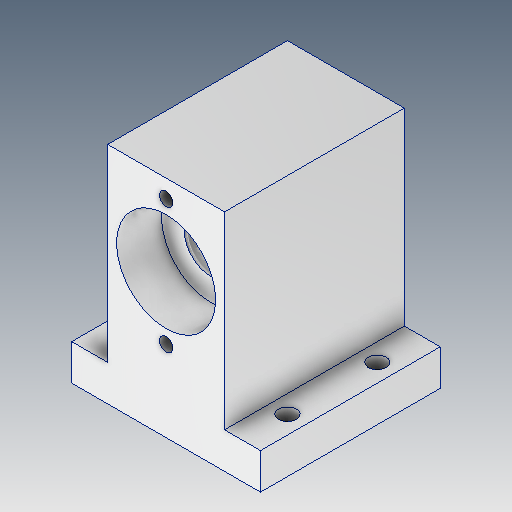
# Autodesk Inventor part: Soporte de tuerca de mesa
Saved by Autodesk Inventor 2020.3 (Build 243373000, 373)
## iProperties
Created: 2020-05-16
Part Number: Soporte de tuerca de mesa
Material: Aluminum 6061
Document SubType Name: Modeling
Designer: Pipi
Density: 2.7 g/cm^3
Appearance: Aluminum - Flat
Mass: 118.391 g
Surface Area: 121.696 cm^2
Volume: 43.8487 cm^3
Author: Pipi
Autodesk Inventor part; units mm, degrees
ref_plane "YZ Plane" through (0, 0, 0) normal (1, 0, 0) x (0, 1, 0)
ref_plane "XZ Plane" through (0, 0, 0) normal (0, 1, 0) x (-1, 0, 0)
ref_plane "XY Plane" through (0, 0, 0) normal (0, 0, 1) x (1, 0, 0)
sketch "Boceto14" plane through (0, 0, 0) normal (0, 1, 0) x (-1, 0, 0)
  line L0 (39.2545, 8.1893) -> (39.2545, -3.9647)
  line L1 (39.2545, -3.9647) -> (39.2545, 20.0353)
  line L2 (31.2545, 22.0353) -> (-2.7455, 22.0353)
  line L3 (-4.7455, -3.9647) -> (31.2545, -3.9647)
  line L4 (39.2545, 20.0353) -> (39.2545, 30.0353)
  line L5 (39.2545, -3.9647) -> (39.2545, -11.9647)
  circle A0 centre (7.2547, 9.0353) radius 11
  line L6 (-2.7455, 22.0353) -> (-8.7455, 22.0353)
  line L7 (-8.7455, -3.9647) -> (-4.7455, -3.9647)
  line L8 (-8.7455, 22.0353) -> (-10.7455, 22.0353)
  line L9 (-10.7455, 22.0353) -> (-10.7455, -3.9647)
  line L10 (-10.7455, -3.9647) -> (-8.7455, -3.9647)
  circle A1 centre (7.2547, 9.0353) radius 6
  line L11 (39.2545, -11.9647) -> (31.2545, -11.9647)
  line L12 (31.2545, -11.9647) -> (31.2545, -3.9647)
  line L13 (39.2545, 30.0353) -> (31.2545, 30.0353)
  line L14 (31.2545, 30.0353) -> (31.2545, 22.0353)
  point P0 (0, 0)
  dimension "d81" = 42
  dimension "d122" = 22
  dimension "d151" = 2
  dimension "d165" = 31.9998
  dimension "d166" = 12
  dimension "d171" = 13
  dimension "d182" = 8
  dimension "d183" = 8
  dimension "d185" = 8
  dimension "d186" = 8
  constraints: 30 end point, 4 perpendicular, 4 point on line, 2 centre point, 2 coincident, 2 horizontal, 2 vertical, 1 collinear, 1 parallel
  measures "d81" distance of L5.end L4.end
  measures "d122" diameter of A0
  measures "d151" distance of L6.end L8.end
  measures "d165" distance from line of L1 A0.centre
  measures "d166" diameter of A1
  measures "d171" distance from line of L3 A0.centre
  measures "d182" distance of L5.end L11.end
  measures "d183" distance of L4.end L13.end
  measures "d185" distance of L11.end L3.end
  measures "d186" distance of L13.end L2.start
extrude "Extrusión14" add sketch "Boceto14" along normal blind 40 contours L0 L5 L11 L12 L3 L7 L10 L9 L8 L6 L2 L14 L13 L4 L1 | A0 | A1
sketch "Boceto23" plane through (0, 0, 0) normal (0, -1, 0) x (1, 0, 0)
  point P0 (0, 0)
hole "Agujero1" at (-7.2547, 0, 9.0353) direction (0, 1, 0) diameter 22 depth 40 tip angle 118
extrude "Extrusión20" add sketch "Boceto14" along normal blind 30 contours A0
sketch "Boceto26" plane through (-39.2545, 0, -11.9647) normal (-1, 0, 0) x (0, 0, 1)
  line L0 (42, 0) -> (42, 40) projected
  line L1 (42, 0) -> (38, 0)
  line L2 (0, 0) -> (42, 0) projected
  line L3 (38, 0) -> (38, 40)
  line L4 (0, 40) -> (42, 40) projected
  line L5 (8, 0) -> (0, 0) projected
  line L6 (0, 0) -> (4, 0)
  line L7 (4, 0) -> (4, 40)
  line L8 (38, 40) -> (38, 30)
  line L9 (38, 30) -> (4, 30)
  line L10 (4, 0) -> (4, 10)
  line L11 (4, 10) -> (38, 10)
  circle A0 centre (38, 10) radius 2
  circle A1 centre (4, 10) radius 2
  circle A2 centre (4, 30) radius 2
  circle A3 centre (38, 30) radius 2
  point P0 (11.9647, 0)
  dimension "d200" = 4
  dimension "d201" = 4
  dimension "d202" = 10
  dimension "d203" = 10
  dimension "d204" = 4
  dimension "d205" = 4
  dimension "d206" = 4
  dimension "d207" = 4
  constraints: 16 end point, 6 point on line, 4 centre point, 4 coincident, 4 perpendicular, 1 midpoint
  measures "d200" distance of L0.start L1.end
  measures "d201" distance of L2.start L6.end
  measures "d202" distance of L3.end L8.end
  measures "d203" distance of L6.end L10.end
  measures "d204" diameter of A0
  measures "d205" diameter of A1
  measures "d206" diameter of A2
  measures "d207" diameter of A3
extrude "Extrusión21" cut sketch "Boceto26" against normal blind 30 contours A0 L11 L3 | L3 A0 | A3 L3 | L3 L9 A3 | L11 A0 L3 | L3 A3 L9 | A2 L9 L7 | L7 A2 | A1 L7 | L7 L11 A1 | L11 L7 A1 | A2 L7 L9
thread "Rosca11" size "M12x1.5" class "6H" standard "ISO Metric profile" length 430
hole "Agujero3" at (-7.2547, 0, 9.0353) direction (0, 1, 0) diameter 14 depth 0.01 tip angle 118
sketch "Boceto27" plane through (0, 40, 0) normal (0, 1, 0) x (1, 0, 0)
  circle A0 centre (-7.2547, -9.0353) radius 6 projected
  line L0 (-7.2547, -9.0353) -> (6.7453, -9.0353)
  line L1 (6.7453, -9.0353) -> (-21.2547, -9.0353)
  circle A1 centre (6.7453, -9.0353) radius 1.5
  circle A2 centre (-21.2547, -9.0353) radius 1.5
  point P0 (0, 0)
  dimension "d226" = 14
  dimension "d227" = 28
  dimension "d228" = 3
  dimension "d229" = 3
  constraints: 4 end point, 2 centre point, 2 coincident, 2 horizontal
  measures "d226" distance of L0.start L0.end
  measures "d227" distance of L0.end L1.end
  measures "d228" diameter of A1
  measures "d229" diameter of A2
hole "Agujero4" at (-21.2547, 40, 9.0353) at (6.7453, 40, 9.0353) direction (0, -1, 0) diameter 3 depth 10 tip angle 118
thread "Rosca12" size "M3x0.5" class "6H" standard "ISO Metric profile" length 7
thread "Rosca13" size "M3x0.5" class "6H" standard "ISO Metric profile" length 7
